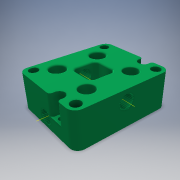
# Autodesk Inventor part: Carro XY_economico
Saved by Autodesk Inventor 2016 (Build 200138000, 138)
## iProperties
Created: 2016-08-10
Part Number: Carro XY_economico
Material: ABS Plastic
Document SubType Name: Modeling
Designer: Waldo
Density: 1.06 g/cm^3
Appearance: Smooth - White
Author: Waldo
Autodesk Inventor part; units mm, degrees
ref_plane "YZ Plane" through (0, 0, 0) normal (1, 0, 0) x (0, 1, 0)
ref_plane "XZ Plane" through (0, 0, 0) normal (0, 1, 0) x (-1, 0, 0)
ref_plane "XY Plane" through (0, 0, 0) normal (0, 0, 1) x (1, 0, 0)
sketch "Sketch1" plane through (0, 0, 0) normal (0, 1, 0) x (-1, 0, 0)
  line L0 (30, 25) -> (-30, 25)
  line L1 (-30, 25) -> (-30, -25)
  line L2 (-30, -25) -> (30, -25)
  line L3 (30, -25) -> (30, 25)
  point P0 (0, 0)
  point P1 (30, 0)
  point P2 (0, -25)
  dimension "d0" = 50
  dimension "d1" = 60
  constraints: 8 end point, 2 midpoint, 2 parallel, 1 horizontal, 1 horizontal alignment, 1 perpendicular, 1 vertical alignment
  measures "d0" distance of L2.end L0.start
  measures "d1" distance of L0.start L0.end
extrude "Extrusion1" add sketch "Sketch1" along normal blind 22
sketch "Sketch2" plane through (30, 0, 25) normal (1, 0, 0) x (0, 0, -1)
  circle A0 centre (25, 6) radius 4.5
  line L0 (0, 0) -> (50, 0) projected
  line L1 (0, 22) -> (50, 22) projected
  point P0 (25, 0)
  point P1 (25, 22)
  dimension "d4" = 9
  dimension "d18" = 6
  constraints: 1 centre point, 1 midpoint, 1 vertical alignment
  measures "d4" diameter of A0
  measures "d18" distance from line of L0 A0.centre
extrude "Extrusion2" cut sketch "Sketch2" against normal through all
sketch "Sketch3" plane through (-30, 0, 25) normal (0, 0, 1) x (1, 0, 0)
  line L0 (72, 6) -> (-12, 6) projected
  circle A0 centre (30, 15) radius 4.5
  line L1 (0, 22) -> (60, 22) projected
  point P0 (30, 0)
  point P1 (30, 22)
  dimension "d7" = 9
  dimension "d8" = 9
  constraints: 1 centre point, 1 midpoint, 1 vertical alignment
  measures "d7" diameter of A0
  measures "d8" distance from line of L0 A0.centre
extrude "Extrusion3" cut sketch "Sketch3" against normal through all
sketch "Sketch4" plane through (30, 0, 25) normal (1, 0, 0) x (0, 0, -1)
  circle A0 centre (25, 6) radius 4.5 projected
  circle A1 centre (25, 6) radius 7.5
  point P0 (25, 0)
  dimension "d11" = 15
  constraints: 1 centre point, 1 coincident
  measures "d11" diameter of A1
extrude "Extrusion4" [suppressed]
fillet "Fillet1" radius 5 4 edges at (30, 11, -25) (30, 11, 25) (-30, 11, -25) (-30, 11, 25)
sketch "Sketch8" plane through (0, 0, 0) normal (0, -1, 0) x (1, 0, 0)
  circle A0 centre (-14, -13) radius 8
  line L0 (25, -25) -> (-25, -25) projected
  line L1 (-30, -20) -> (-30, 20) projected
  point P0 (0, 0)
  dimension "d25" = 16
  dimension "d26" = 12
  dimension "d27" = 16
  constraints: 1 centre point
  measures "d25" diameter of A0
  measures "d26" distance from line of A0.centre L0
  measures "d27" distance from line of L1 A0.centre
extrude "Extrusion8" cut sketch "Sketch8" against normal blind 4
sketch "Sketch9" plane through (-14, 4, -13) normal (0, -1, 0) x (1, 0, 0)
  circle A0 centre (0, 0) radius 8 projected
  point P0 (14, 13)
  constraints: 1 coincident
hole "Hole1" at (-14, 4, -13) direction (0, 1, 0) diameter 2 end through all
sketch "Sketch10" plane through (0, 0, 0) normal (0, -1, 0) x (1, 0, 0)
  circle A0 centre (-13.5, 13.5) radius 5
  circle A1 centre (-14, -13) radius 8 construction
  line L0 (30, 4.5) -> (-30, 4.5) projected
  line L1 (-4.5, 25) -> (-4.5, -25) projected
  point P0 (0, 0)
  point P1 (-13.5, 8.5)
  point P2 (-8.5, 13.5)
  dimension "d39" = 10
  dimension "d88" = 4
  dimension "d89" = 4
  constraints: 2 point on circle, 1 centre point, 1 horizontal alignment, 1 vertical alignment
  measures "d39" diameter of A0
  measures "d88" distance from line of L0 A0.start
  measures "d89" distance from line of L1 A0.end
extrude "Extrusion9" cut sketch "Sketch10" against normal through all
mirror "Mirror3" about plane through (0, 0, 0) normal (1, 0, 0) of "Extrusion9", "Extrusion8", "Hole1"
fillet "Fillet3" radius 1 4 edges at (18.5, 22, 13.5) (-18.5, 22, 13.5) (18.5, 0, 13.5) (-18.5, 0, 13.5)
sketch "Sketch11" plane through (0, 22, 0) normal (0, 1, 0) x (1, 0, 0)
  circle A0 centre (14, 13) radius 1 projected
  circle A1 centre (-14, 13) radius 1 projected
  circle A2 centre (-14, 13) radius 4.6
  circle A3 centre (14, 13) radius 1 projected
  circle A4 centre (14, 13) radius 4.6
  point P0 (0, 0)
  dimension "d44" = 9.2
  dimension "d45" = 9.2
  constraints: 2 centre point, 2 coincident
  measures "d44" diameter of A2
  measures "d45" diameter of A4
extrude "Extrusion10" cut sketch "Sketch11" against normal blind 6
fillet "Fillet4" radius 0.5 2 edges at (9.4, 22, -13) (-18.6, 22, -13)
sketch "Sketch12" plane through (0, 0, 0) normal (0, -1, 0) x (1, 0, 0)
  line L0 (-30, -20) -> (-30, 20) projected
  line L1 (30, 20) -> (30, -20) projected
  line L2 (25, -25) -> (-25, -25) projected
  line L3 (30, -4.5) -> (-30, -4.5) projected
  line L4 (-4.5, 25) -> (-4.5, -25) projected
  point P0 (0, 0)
  point P1 (-25, -20)
  point P2 (25, -20)
  point P3 (-27, -9.5)
  point P4 (27, -9.5)
  point P5 (24, 20)
  point P6 (-24, 20)
  point P7 (-30, 0)
  point P8 (30, 0)
  dimension "d49" = 20
  dimension "d50" = 24
  dimension "d51" = 24
  dimension "d53" = 3
  dimension "d54" = 3
  dimension "d55" = 5
  dimension "d56" = 5
  dimension "d57" = 5
  dimension "d90" = 5
  constraints: 3 horizontal alignment
  measures "d49" vertical distance of point (0, 0) point (-24, 20)
  measures "d50" horizontal distance of point (0, 0) point (-24, 20)
  measures "d51" horizontal distance of point (24, 20) point (0, 0)
  measures "d53" distance from line of L0 point (-27, -9.5)
  measures "d54" distance from line of L1 point (27, -9.5)
  measures "d55" distance from line of L0 point (-25, -20)
  measures "d56" distance from line of L2 point (-25, -20)
  measures "d57" distance from line of L1 point (25, -20)
  measures "d90" distance from line of point (-27, -9.5) L3
hole "Hole2" at (-25, 0, -20) at (25, 0, -20) at (-27, 0, -9.5) at (27, 0, -9.5) at (24, 0, 20) at (-24, 0, 20) direction (0, 1, 0) diameter 3 end through all
sketch "Sketch13" plane through (0, 22, 0) normal (0, 1, 0) x (1, 0, 0)
  circle A0 centre (24, -20) radius 1.5 projected
  circle A1 centre (-27, 9.5) radius 1.5 projected
  circle A2 centre (-25, 20) radius 1.5 projected
  circle A3 centre (25, 20) radius 1.5 projected
  circle A4 centre (27, 9.5) radius 1.5 projected
  circle A5 centre (-24, -20) radius 1.5 projected
  circle A6 centre (14, 13) radius 5.1 projected
  circle A7 centre (13.5, -13.5) radius 6 projected
  arc A8 (-30, -20) -> (-25, -25) centre (-25, -20) ccw projected
  line L0 (-25, -25) -> (25, -25) projected
  arc A9 (25, -25) -> (30, -20) centre (25, -20) ccw projected
  line L1 (30, -20) -> (30, 20) projected
  arc A10 (30, 20) -> (25, 25) centre (25, 20) ccw projected
  line L2 (25, 25) -> (-25, 25) projected
  arc A11 (-25, 25) -> (-30, 20) centre (-25, 20) ccw projected
  line L3 (-30, 20) -> (-30, -20) projected
  circle A12 centre (-13.5, -13.5) radius 6 projected
  circle A13 centre (-14, 13) radius 5.1 projected
  point P0 (0, 0)
  constraints: 6 coincident
sketch "Sketch14" plane through (0, 22, 0) normal (0, 1, 0) x (1, 0, 0)
  circle A0 centre (27, 9.5) radius 1.5 projected
  circle A1 centre (-27, 9.5) radius 1.5 projected
  point P0 (0, 0)
  constraints: 2 coincident
hole "Hole4" at (27, 22, -9.5) at (-27, 22, -9.5) direction (0, -1, 0) diameter 7 depth 13
hole "Hole5" at (24, 22, 20) at (25, 22, -20) at (-25, 22, -20) at (-24, 22, 20) direction (0, -1, 0) diameter 6 depth 19
fillet "Fillet6" radius 2 4 edges at (30, 15.5, -11.3028) (30, 15.5, -7.6972) (-30, 15.5, -7.6972) (-30, 15.5, -11.3028)
sketch "Sketch15" plane through (25, 0, -25) normal (0, 0, -1) x (-1, 0, 0)
  circle A0 centre (25, 15) radius 4.5 projected
  arc A1 (25.2172, 19.1443) -> (24.7828, 19.1443) centre (25, 15) ccw
  line L0 (24.7645, 19.4938) -> (24.7828, 19.1443)
  line L1 (25.2355, 19.4938) -> (25.2172, 19.1443)
  line L2 (25, 15) -> (25, 25.9123) construction
  line L3 (25.2172, 19.1443) -> (25, 15) construction
  line L4 (25, 15) -> (24.7828, 19.1443) construction
  arc A2 (25.2355, 19.4938) -> (24.7645, 19.4938) centre (25, 15) ccw construction
  point P0 (25, 0)
  dimension "d91" = 8.3
  dimension "d92" = 3
  dimension "d93" = 3
  constraints: 10 end point, 6 point on circle, 2 centre point, 2 collinear, 2 line through centre, 1 coincident, 1 concentric, 1 vertical
  measures "d91" diameter of A1
  measures "d92" angle of L2 L1
  measures "d93" angle of L0 L2
extrude "Extrusion11" add sketch "Sketch15" against normal blind 15 contours L1 A1 L0 A0 picked at (24.9759, 19.3827)
pattern_circular "Circular Pattern1" count 30 over 360 about axis through (0, 15, 25) along (0, 0, -1) of "Extrusion11"
mirror "Mirror4" about plane through (0, 0, 0) normal (0, 0, 1) of "Extrusion11", "Circular Pattern1"
sketch "Sketch16" plane through (-30, 0, -20) normal (-1, 0, 0) x (0, 0, 1)
  circle A0 centre (20, 6) radius 4.5 projected
  arc A1 (20.2172, 10.1443) -> (19.7828, 10.1443) centre (20, 6) ccw
  line L0 (20, 6) -> (20, 12.6683) construction
  line L1 (20.2355, 10.4938) -> (20.2172, 10.1443)
  line L2 (19.7645, 10.4938) -> (19.7828, 10.1443)
  line L3 (20, 6) -> (20.2172, 10.1443) construction
  line L4 (20, 6) -> (19.7828, 10.1443) construction
  arc A2 (19.7645, 10.4938) -> (20.2355, 10.4938) centre (20, 6) ccw
  point P0 (20, 0)
  dimension "d99" = 8.3
  dimension "d100" = 3
  dimension "d101" = 3
  constraints: 10 end point, 7 point on circle, 2 centre point, 2 collinear, 2 line through centre, 1 coincident, 1 vertical
  measures "d99" diameter of A1
  measures "d100" angle of L0 L1
  measures "d101" angle of L2 L0
extrude "Extrusion12" add sketch "Sketch16" against normal blind 15 contours L1 A1 L2 A0 picked at (19.9759, 10.3827)
pattern_circular "Circular Pattern2" count 30 over 360 about axis through (30, 6, 0) along (-1, 0, 0) of "Extrusion12"
mirror "Mirror5" about plane through (0, 0, 0) normal (1, 0, 0) of "Extrusion12", "Circular Pattern2"
sketch "Sketch17" plane through (0, 22, 0) normal (0, 1, 0) x (1, 0, 0)
  line L0 (8, -6) -> (8, 6)
  line L1 (8, 6) -> (6, 8)
  line L2 (6, 8) -> (-6, 8)
  line L3 (-6, 8) -> (-8, 6)
  line L4 (-8, 6) -> (-8, -6)
  line L5 (-8, -6) -> (-6, -8)
  line L6 (-6, -8) -> (6, -8)
  line L7 (6, -8) -> (8, -6)
  point P0 (0, 0)
  point P1 (-8, 0)
  point P2 (8, 0)
  point P3 (0, -8)
  point P4 (0, 8)
  dimension "d107" = 12
  dimension "d108" = 12
  dimension "d109" = 12
  dimension "d110" = 12
  dimension "d111" = 8
  dimension "d112" = 8
  dimension "d113" = 8
  constraints: 16 end point, 4 midpoint, 3 parallel, 2 horizontal alignment, 2 vertical alignment, 1 perpendicular, 1 vertical
  measures "d107" distance of L5.end L6.end
  measures "d108" distance of L3.end L4.end
  measures "d109" distance of L1.end L2.end
  measures "d110" distance of L0.start L0.end
  measures "d111" distance from line of point (0, 0) L2
  measures "d112" distance from line of point (0, 0) L6
  measures "d113" distance from line of point (0, 0) L0
extrude "Extrusion13" cut sketch "Sketch17" against normal through all
fillet "Fillet7" radius 1 8 edges at (7, 22, -7) (8, 22, 0) (7, 22, 7) (0, 22, 8) (-7, 22, 7) (-8, 22, 0) (-7, 22, -7) (0, 22, -8)
fillet "Fillet8" radius 2 16 edges at (-6.1213, 21.7071, 8.2929) (-6, 10.5, 8) (-8.2929, 21.7071, 6.1213) (-8, 10.5, 6) (-8.2929, 21.7071, -6.1213) (-8, 10.5, -6) (-6.1213, 21.7071, -8.2929) (-6, 10.5, -8) (6.1213, 21.7071, 8.2929) (6, 10.5, 8) (8.2929, 21.7071, 6.1213) (8, 10.5, 6) (6.1213, 21.7071, -8.2929) (6, 10.5, -8) (8.2929, 21.7071, -6.1213) (8, 10.5, -6)
equation "\"d45\" = d44"
equation "\"d51\" = d50"
equation "\"d53\" = d54"
equation "\"d55\" = d57"
equation "\"d93\" = d92"
equation "\"d101\" = d100"
equation "\"d108\" = d107"
equation "\"d109\" = d107"
equation "\"d110\" = d107"
equation "\"d112\" = d111"
body "Solid1"
